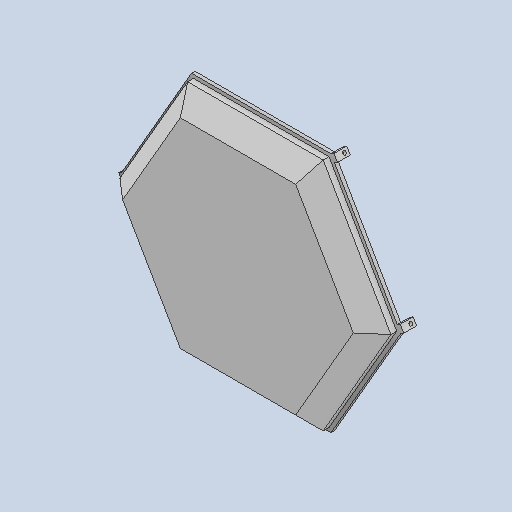
# Autodesk Inventor part: tapaHEX
Saved by Autodesk Inventor 2024 (Build 280153000, 153)
## iProperties
Created: 2024-03-21
Part Number: tapaHEX
Material: Genérico
Document SubType Name: Modeling
Designer: na_re
Density: 1 g/cm^3
Appearance: Valor por defecto
Author: na_re
Autodesk Inventor part; units mm, degrees
ref_plane "YZ Plane" through (0, 0, 0) normal (1, 0, 0) x (0, 1, 0)
ref_plane "XZ Plane" through (0, 0, 0) normal (0, 1, 0) x (-1, 0, 0)
ref_plane "XY Plane" through (0, 0, 0) normal (0, 0, 1) x (1, 0, 0)
ref_plane "Plano de trabajo1" through (0, 0, 0) normal (0, 0, 1) x (1, 0, 0)
sketch "Boceto1" plane through (0, 0, 0) normal (0, 0, 1) x (1, 0, 0)
  line L0 (58.8453, 101.923) -> (-58.8453, 101.923) projected
  line L1 (-58.8453, 101.923) -> (-117.6906, 0) projected
  line L2 (-117.6906, 0) -> (-58.8453, -101.923) projected
  line L3 (-58.8453, -101.923) -> (58.8453, -101.923) projected
  line L4 (58.8453, -101.923) -> (117.6906, 0) projected
  line L5 (117.6906, 0) -> (58.8453, 101.923) projected
  line L6 (-60, 103.923) -> (-120, 0) projected
  line L7 (-120, 0) -> (-60, -103.923) projected
  line L8 (-60, -103.923) -> (60, -103.923) projected
  line L9 (60, -103.923) -> (120, 0) projected
  line L10 (120, 0) -> (60, 103.923) projected
  line L11 (60, 103.923) -> (-60, 103.923) projected
  line L12 (58.8453, 101.923) -> (117.6906, 0) projected
  line L13 (117.6906, 0) -> (58.8453, -101.923) projected
  line L14 (58.8453, -101.923) -> (-58.8453, -101.923) projected
  line L15 (-58.8453, -101.923) -> (-117.6906, 0) projected
  line L16 (-117.6906, 0) -> (-58.8453, 101.923) projected
  line L17 (-58.8453, 101.923) -> (58.8453, 101.923) projected
  point P0 (0, 0)
extrude "Extrusión1" add sketch "Boceto1" along normal blind 3 contours L5 L4 L3 L2 L1 L0 | L11 L10 L9 L8 L7 L6
sketch "Boceto2" plane through (0, 0, 3) normal (0, 0, 1) x (1, 0, 0)
  line L0 (-120, 0) -> (-60, -103.923) projected
  line L1 (-60, -103.923) -> (60, -103.923) projected
  line L2 (60, -103.923) -> (120, 0) projected
  line L3 (120, 0) -> (60, 103.923) projected
  line L4 (60, 103.923) -> (-60, 103.923) projected
  line L5 (-60, 103.923) -> (-120, 0) projected
  line L6 (58.2679, 100.923) -> (116.5359, 0)
  line L7 (116.5359, 0) -> (58.2679, -100.923)
  line L8 (58.2679, -100.923) -> (-58.2679, -100.923)
  line L9 (-58.2679, -100.923) -> (-116.5359, 0)
  line L10 (-116.5359, 0) -> (-58.2679, 100.923)
  line L11 (-58.2679, 100.923) -> (58.2679, 100.923)
  point P0 (0, 0)
  dimension "d2" = 3
  constraints: 12 end point, 5 other
  measures "d2" distance between parallel lines of L3 L6
extrude "Extrusión2" add sketch "Boceto2" along normal blind 20 contours L6 L7 L8 L9 L10 L11
chamfer "Chaflán1" distance 15 angle 45 6 edges at (-87.4019, 50.4615, 23) (-87.4019, -50.4615, 23) (0, -100.923, 23) (87.4019, -50.4615, 23) (87.4019, 50.4615, 23) (0, 100.923, 23)
sketch "Boceto3" plane through (0, 0, 0) normal (0, 0, -1) x (-1, 0, 0)
  line L0 (117.6906, 0) -> (58.8453, -101.923) projected
  line L1 (58.8453, -101.923) -> (-58.8453, -101.923) projected
  line L2 (58.8453, 101.923) -> (117.6906, 0) projected
  line L3 (-117.6906, 0) -> (-58.8453, 101.923) projected
  line L4 (-58.8453, -101.923) -> (-117.6906, 0) projected
  point P0 (0, 0)
shell "Vaciado1" thickness 3 removed faces 1 at (-20, 34.641, 0)
sketch "Boceto4" plane through (-60, -103.923, 0) normal (-0.866, -0.5, 0) x (0, 0, 1)
  line L0 (0, 120) -> (0, 0) projected
  line L1 (0, 0) -> (3, 0) projected
  line L2 (3, 120) -> (3, 0) projected
  line L3 (0, 120) -> (3, 120) projected
  line L4 (0, 120) -> (3, 120) projected
  line L5 (0, 0) -> (0, 120) projected
  line L6 (3, 120) -> (0, 120)
  line L7 (0, 120) -> (0, 114)
  line L8 (0, 114) -> (3, 114)
  line L9 (3, 114) -> (3, 120)
  line L10 (0, 0) -> (3, 0)
  line L11 (3, 0) -> (3, 6)
  line L12 (3, 6) -> (0, 6)
  line L13 (0, 6) -> (0, 0)
  point P0 (0, 60)
  point P1 (0, 114)
  point P2 (3, 114)
  point P3 (0, 6)
  dimension "d9" = 6
  dimension "d10" = 6
  constraints: 16 end point, 4 parallel, 2 horizontal, 2 perpendicular, 2 point on line
  measures "d9" distance of L7.end L6.end
  measures "d10" distance of L11.end L10.end
extrude "Extrusión3" add sketch "Boceto4" along normal blind 3 contours L3 L2 L8 L0 | L12 L2 L1 L0
sketch "Boceto5" plane through (0, 0, 0) normal (0, 0, -1) x (-1, 0, 0)
  line L0 (-56.5359, 97.923) -> (56.5359, 97.923) projected
  line L1 (56.5359, 97.923) -> (113.0718, 0) projected
  line L2 (113.0718, 0) -> (56.5359, -97.923) projected
  line L3 (56.5359, -97.923) -> (-56.5359, -97.923) projected
  line L4 (-56.5359, -97.923) -> (-113.0718, 0) projected
  line L5 (-113.0718, 0) -> (-56.5359, 97.923) projected
  line L6 (60, 103.923) -> (120, 0) projected
  line L7 (-60, 103.923) -> (60, 103.923) projected
  line L8 (-120, 0) -> (-60, 103.923) projected
  line L9 (-60, -103.923) -> (-120, 0) projected
  line L10 (60, -103.923) -> (-60, -103.923) projected
  line L11 (60, -103.923) -> (62.5981, -105.423) projected
  line L12 (65.5981, -100.2269) -> (62.5981, -105.423) projected
  line L13 (63, -98.7269) -> (65.5981, -100.2269) projected
  line L14 (117, -5.1962) -> (63, -98.7269) projected
  line L15 (117, -5.1962) -> (119.5981, -6.6962) projected
  line L16 (122.5981, -1.5) -> (119.5981, -6.6962) projected
  line L17 (120, 0) -> (122.5981, -1.5) projected
  line L18 (120, 0) -> (117, -5.1962)
  line L19 (63, -98.7269) -> (60, -103.923)
  point P0 (0, 0)
  constraints: 4 end point, 1 perpendicular
extrude "Extrusión4" add sketch "Boceto5" along normal blind 8 contours L17 L16 L15 L18 | L13 L12 L11 L19
sketch "Boceto6" plane through (-62.5981, -105.423, 0) normal (-0.866, -0.5, 0) x (0, 0, 1)
  line L0 (3, 114) -> (-8, 114) projected
  line L1 (-8, 114) -> (-8, 117)
  line L2 (-8, 114) -> (-8, 120) projected
  line L3 (-8, 117) -> (-4.5, 117)
  circle A0 centre (-4.5, 117) radius 1.5
  line L4 (-8, 6) -> (-8, 0) projected
  line L5 (-8, 6) -> (-8, 3)
  line L6 (-8, 3) -> (-4.5, 3)
  circle A1 centre (-4.5, 3) radius 1.5
  point P0 (0, 60)
  dimension "d15" = 3.5
  dimension "d16" = 3
  dimension "d17" = 3.5
  dimension "d18" = 3
  constraints: 8 end point, 2 centre point, 2 coincident, 2 midpoint, 2 perpendicular
  measures "d15" distance of L1.end L3.end
  measures "d16" diameter of A0
  measures "d17" distance of L5.end L6.end
  measures "d18" diameter of A1
extrude "Extrusión5" cut sketch "Boceto6" against normal blind 8
sketch "Boceto7" plane through (60, 103.923, 3) normal (0.866, 0.5, 0) x (0, 0, -1)
  line L0 (3, -120) -> (3, 0) projected
  line L1 (3, 0) -> (0, 0) projected
  line L2 (0, -120) -> (0, 0) projected
  line L3 (3, -120) -> (0, -120) projected
  line L4 (3, -120) -> (0, -120)
  line L5 (0, -120) -> (0, -114)
  line L6 (0, -114) -> (3, -114)
  line L7 (3, -114) -> (3, -120)
  line L8 (3, 0) -> (0, 0)
  line L9 (0, 0) -> (0, -6)
  line L10 (0, -6) -> (3, -6)
  line L11 (3, -6) -> (3, 0)
  point P0 (3, -60)
  point P1 (3, -114)
  point P2 (3, -6)
  dimension "d21" = 6
  dimension "d22" = 6
  constraints: 16 end point, 4 parallel, 2 horizontal, 2 perpendicular, 2 point on line
  measures "d21" distance of L4.end L5.end
  measures "d22" distance of L9.end L8.end
extrude "Extrusión6" add sketch "Boceto7" along normal blind 3 contours L3 L2 L6 L0 | L10 L2 L1 L0
sketch "Boceto8" plane through (0, 0, 0) normal (0, 0, -1) x (-1, 0, 0)
  line L0 (-56.5359, 97.923) -> (56.5359, 97.923) projected
  line L1 (56.5359, 97.923) -> (113.0718, 0) projected
  line L2 (113.0718, 0) -> (56.5359, -97.923) projected
  line L3 (56.5359, -97.923) -> (-56.5359, -97.923) projected
  line L4 (-56.5359, -97.923) -> (-113.0718, 0) projected
  line L5 (-113.0718, 0) -> (-56.5359, 97.923) projected
  line L6 (60, -103.923) -> (63, -98.7269) projected
  line L7 (117, -5.1962) -> (63, -98.7269) projected
  line L8 (117, -5.1962) -> (120, 0) projected
  line L9 (60, 103.923) -> (120, 0) projected
  line L10 (-60, 103.923) -> (60, 103.923) projected
  line L11 (-60, 103.923) -> (-62.5981, 105.423) projected
  line L12 (-65.5981, 100.2269) -> (-62.5981, 105.423) projected
  line L13 (-63, 98.7269) -> (-65.5981, 100.2269) projected
  line L14 (-117, 5.1962) -> (-63, 98.7269) projected
  line L15 (-117, 5.1962) -> (-119.5981, 6.6962) projected
  line L16 (-122.5981, 1.5) -> (-119.5981, 6.6962) projected
  line L17 (-120, 0) -> (-122.5981, 1.5) projected
  line L18 (-60, -103.923) -> (-120, 0) projected
  line L19 (60, -103.923) -> (-60, -103.923) projected
  line L20 (-120, 0) -> (-60, 103.923)
  point P0 (0, 0)
  point P1 (-63, 98.7269)
  point P2 (-117, 5.1962)
  constraints: 2 end point
extrude "Extrusión7" add sketch "Boceto8" along normal blind 8 contours L17 L16 L15 L20 | L13 L12 L11 L20
sketch "Boceto9" plane through (62.5981, 105.423, 3) normal (0.866, 0.5, 0) x (0, 0, -1)
  circle A0 centre (7.5, -117) radius 1.5 projected
  circle A1 centre (7.5, -3) radius 1.5 projected
  point P0 (3, -60)
extrude "Extrusión8" cut sketch "Boceto9" against normal blind 8
